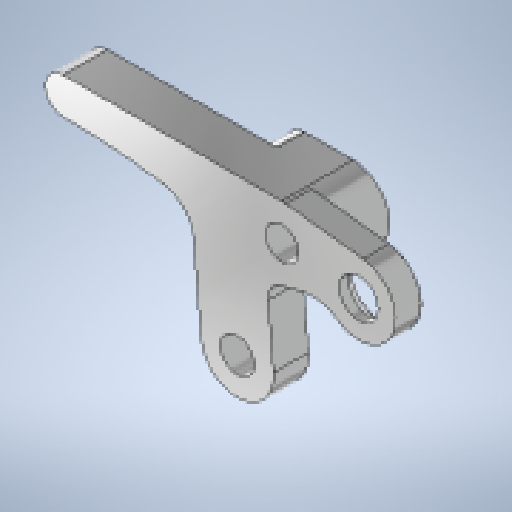
# Autodesk Inventor part: Lever
Saved by Autodesk Inventor 2023.4 (Build 274418000, 418)
## iProperties
Created: 2024-02-17
Part Number: Lever
Material: Aluminum 6061
Document SubType Name: Modeling
Designer: Nathan Cai
Density: 2.7 g/cm^3
Appearance: Aluminum - Flat
Arm_Length: 0.438 in
Arm_Angle: 102.50 deg
Author: Nathan Cai
Autodesk Inventor part; units mm, degrees
ref_plane "YZ Plane" through (0, 0, 0) normal (1, 0, 0) x (0, 1, 0)
ref_plane "XZ Plane" through (0, 0, 0) normal (0, 1, 0) x (-1, 0, 0)
ref_plane "XY Plane" through (0, 0, 0) normal (0, 0, 1) x (1, 0, 0)
sketch "Sketch1" plane through (0, 0, 0) normal (0, 0, 1) x (1, 0, 0)
  circle A0 centre (0, 0) radius 1.4224
  circle A1 centre (0, 0) radius 3.175
  line L0 (0, 0) -> (-19.05, 0) construction
  circle A2 centre (-2.4765, -10.833) radius 3.175
  circle A3 centre (-2.4765, -10.833) radius 5 construction
  circle A4 centre (-2.4765, -10.833) radius 1.5
  line L1 (0, 0) -> (-2.4765, -10.833) construction
  line L2 (-2.4765, -10.833) -> (-3.9388, -10.4987) construction
  line L3 (0, 0) -> (-2.4765, -10.833) construction
  arc A5 (-5.5433, -10.0113) -> (0.5903, -11.6548) centre (-2.4765, -10.833) ccw
  arc A6 (-1.0297, -3.0034) -> (-19.05, 0) centre (-19.05, -55.5625) ccw
  arc A7 (-19.05, 3.175) -> (-19.05, 0) centre (-19.05, 1.5875) ccw
  line L4 (-19.05, 3.175) -> (0, 3.175)
  line L5 (-2.4765, -10.833) -> (-4.8781, 0) construction
  line L6 (0.6232, -10.1458) -> (-1.7784, 0.6872)
  line L7 (-7.9779, -0.6872) -> (-5.5762, -11.5202)
  arc A8 (-5.5762, -11.5202) -> (0.6232, -10.1458) centre (-2.4765, -10.833) ccw
  arc A9 (-1.7784, 0.6872) -> (-7.9779, -0.6872) centre (-4.8781, 0) ccw
  circle A10 centre (6.7469, -0.7937) radius 3.175
  circle A11 centre (6.7469, -0.7937) radius 1.5
  line L8 (7.1178, 2.3595) -> (0.371, 3.1533)
  arc A12 (4.7206, -3.2381) -> (-0.2367, -6.2667) centre (2.7611, -5.6021) ccw
  circle A13 centre (6.7469, -0.7937) radius 5 construction
  point P0 (0.5903, -11.6548)
  point P1 (0, 3.175)
  point P2 (-7.8787, -1.1346)
  point P3 (0.6232, -10.1458)
  point P4 (-0.9547, -3.0281)
  point P5 (-2.4391, 2.0326)
  point P6 (1.2353, -2.9248)
  point P7 (1.4036, -2.8479)
  point P8 (-1.4243, -1.0642)
  point P9 (-1.7024, 0.5129)
  point P10 (0.6232, -10.1458)
  point P11 (-5.5762, -11.5202)
  dimension "d24" = 3
  dimension "d0" = 2.8448
  dimension "d1" = 6.35
  dimension "d9" = 19.05
  dimension "d22" = 6.35
  dimension "d23" = 10
  dimension "Arm_Length" = 11.1125
  dimension "d29" = 3.175
  dimension "d30" = 6.35
  dimension "d31" = 6.35
  dimension "d32" = 3
  dimension "d36" = 10
  dimension "Arm_Angle" = 102.5
  dimension "d38" = 4.7625
  dimension "d39" = 6.7469
  dimension "d40" = 0.7937
  constraints: 22 end point, 17 point on circle, 14 tangent, 13 centre point, 6 coincident, 2 point on line, 1 concentric, 1 horizontal, 1 parallel, 1 perpendicular, 3 other
  measures "d0" diameter of A0
  measures "d1" diameter of A1
  measures "d9" distance of L0.start L0.end
  measures "d22" diameter of A2
  measures "d23" diameter of A3
  measures "Arm_Length" distance from line of point (0, 0) L2
  measures "d29" diameter of A7
  measures "d30" diameter of A9
  measures "d31" diameter of A10
  measures "d32" diameter of A11
  measures "d36" diameter of A13
  measures "Arm_Angle" angle of L0 L5
  measures "d38" distance from line of A0.centre L5
  measures "d39" horizontal distance of A0.centre A11.centre
  measures "d40" vertical distance of A0.centre A11.centre
extrude "Extrusion1" add sketch "Sketch1" along normal blind 3.048 contours A1 L6 A9 | A1 L8 A10 A12 | A1 A9 L4 | A10 | L6 A2 L7 A6 A1 | A1 A9 L6 | A1 A6 L7 A9 | A9 L7 A6 A7 L4 | A2
fillet "Fillet1" radius 3.175 1 edges at (-7.8787, -1.1346, 1.524)
sketch "Sketch2" plane through (0, 0, 0) normal (0, 0, -1) x (-1, 0, 0)
  line L0 (0, 3.175) -> (19.05, 3.175) projected
  arc A0 (0, 3.175) -> (-0.371, 3.1533) centre (0, 0) ccw projected
  line L1 (-7.1178, 2.3595) -> (-0.371, 3.1533) projected
  arc A1 (-7.1178, 2.3595) -> (-4.7206, -3.2381) centre (-6.7469, -0.7937) ccw projected
  arc A2 (-1.4036, -2.8479) -> (-4.7206, -3.2381) centre (-2.7611, -5.6021) ccw projected
  line L2 (-0.6232, -10.1458) -> (0.9547, -3.0281) projected
  arc A3 (-0.6232, -10.1458) -> (5.5762, -11.5202) centre (2.4765, -10.833) ccw projected
  line L3 (7.4238, -3.1863) -> (5.5762, -11.5202) projected
  arc A4 (10.0068, -0.7409) -> (7.4238, -3.1863) centre (10.5236, -3.8735) ccw projected
  arc A5 (19.05, 0) -> (10.0068, -0.7409) centre (19.05, -55.5625) ccw projected
  arc A6 (19.05, 0) -> (19.05, 3.175) centre (19.05, 1.5875) ccw projected
  circle A7 centre (0, 0) radius 1.4224 projected
  circle A8 centre (2.4765, -10.833) radius 1.5 projected
  circle A9 centre (-6.7469, -0.7937) radius 1.5 projected
  line L4 (-7.1178, 2.3595) -> (-0.371, 3.1533) projected
  arc A10 (0, 3.175) -> (-1.4036, -2.8479) centre (0, 0) ccw
  arc A11 (6.5483, -7.1357) -> (0.3488, -5.7613) centre (2.4765, -10.833) ccw
  line L5 (0, 3.175) -> (19.05, 3.175) projected
  arc A12 (10.0068, -0.7409) -> (7.4238, -3.1863) centre (10.5236, -3.8735) ccw projected
  arc A13 (5.7158, 3.175) -> (7.4238, -3.1863) centre (18.4158, 3.175) ccw
  line L6 (0, 3.175) -> (19.05, 3.175) projected
  arc A14 (-1.4036, -2.8479) -> (0.9547, -3.0281) centre (0, 0) ccw projected
  point P0 (0.5325, -5.7729)
  point P1 (6.8533, -6.8432)
  point P2 (0.5998, -5.7406)
  point P3 (-1.4036, -2.8479)
  dimension "d41" = 11
  dimension "d42" = 12.7
  constraints: 8 point on circle, 3 centre point, 3 coincident, 3 point on line, 1 end point, 1 line through centre
  measures "d41" diameter of A11
  measures "d42" radius of A13
extrude "Extrusion2" add sketch "Sketch2" along normal blind 0.7937 contours L0 A13 L3 A11 L2 A14 A10 A0
extrude "Extrusion3" add sketch "Sketch2" along normal blind 3.175 contours L0 A13 L3 A11 L2 A14 A10 A0
fillet "Fillet2" radius 1.5875 6 edges at (-0.3488, -5.7613, -1.5875) (-0.9547, -3.0281, 1.1271) (-0.9547, -3.0281, -1.9844) (-6.5483, -7.1357, -1.5875) (-7.4238, -3.1863, -1.5875) (-5.7158, 3.175, -1.5875)
extrude "Extrusion4" cut sketch "Sketch2" against normal blind 0.7937 contours A10 A2 A1 L1
sketch "Sketch3" plane through (0, 0, 0.7937) normal (0, 0, -1) x (-1, 0, 0)
  circle A0 centre (-6.7469, -0.7937) radius 1.5 projected
  point P0 (0, 0)
  constraints: 1 coincident
hole "Hole2" at (6.7469, -0.7937, 0.7937) direction (0, 0, 1) diameter 3.4036 end through all countersink diameter 6.2992 countersink angle 90 clearance for "Flat Head Machine Screw" size "M3" standard "Ansi Metric M Profile"
body "Solid1"
